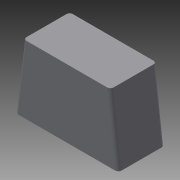
# Autodesk Inventor part: Box MKIV Version 2
Saved by Autodesk Inventor 2013 (Build 170138000, 138)
## iProperties
Created: 2014-12-24
Part Number: Box MKIV Version 2
Material: Generic
Document SubType Name: Modeling
Designer: Zep
Density: 1 g/cm^3
Author: Zep
Autodesk Inventor part; units mm, degrees
ref_plane "YZ Plane" through (0, 0, 0) normal (1, 0, 0) x (0, 1, 0)
ref_plane "XZ Plane" through (0, 0, 0) normal (0, 1, 0) x (-1, 0, 0)
ref_plane "XY Plane" through (0, 0, 0) normal (0, 0, 1) x (1, 0, 0)
sketch "Sketch1" plane through (0, 0, 0) normal (0, 0, 1) x (1, 0, 0)
  line L0 (0, 0) -> (129, 0)
  line L1 (129, 0) -> (129, 85)
  line L2 (129, 85) -> (0, 85)
  line L3 (0, 85) -> (0, 0)
  line L4 (0, 85) -> (10, 85)
  line L5 (10, 85) -> (0, 0)
  line L6 (129, 85) -> (119, 85)
  line L7 (119, 85) -> (129, 0)
  dimension "d0" = 129
  dimension "d1" = 85
  dimension "d2" = 10
  dimension "d3" = 10
  constraints: 16 end point, 2 parallel, 2 point on line, 1 horizontal, 1 perpendicular
  measures "d0" distance of L2.end L1.end
  measures "d1" distance of L1.end L0.end
  measures "d2" distance of L2.end L4.end
  measures "d3" distance of L1.end L6.end
extrude "Extrusion1" add sketch "Sketch1" against normal blind 58 contours L5 L2 L7 L0
fillet "Fillet1" radius 4 4 edges at (5, 42.5, 0) (124, 42.5, 0) (124, 42.5, -58) (5, 42.5, -58)
shell "Shell1" thickness 3 removed faces 1 at (44.3425, 0, -19.3333)
sketch "Sketch3" plane through (0, 0, -58) normal (0, 0, -1) x (-1, 0, 0)
  line L0 (-14.0276, 85) -> (-114.9724, 85) projected
  line L1 (-124.9724, 0) -> (-4.0276, 0) projected
  line L2 (-64.5, 0) -> (-64.5, 85)
  line L3 (-64.5, 85) -> (-64.5, 55)
  circle A0 centre (-64.5, 55) radius 22.5
  line L4 (-64.5, 0) -> (-102.5, 0)
  line L5 (-102.5, 0) -> (-102.5, 20)
  line L6 (-102.5, 20) -> (-64.5, 20)
  line L7 (-64.5, 20) -> (-64.5, 0)
  line L8 (-64.5, 0) -> (-26.5, 0)
  line L9 (-26.5, 0) -> (-26.5, 20)
  line L10 (-26.5, 20) -> (-64.5, 20)
  line L11 (-64.5, 20) -> (-64.5, 0)
  circle A1 centre (-26.5, 20) radius 7.85
  circle A2 centre (-102.5, 20) radius 7.85
  point P0 (0, 0)
  dimension "d18" = 30
  dimension "d19" = 45
  dimension "d20" = 38
  dimension "d21" = 20
  dimension "d22" = 38
  dimension "d23" = 15.7
  dimension "d24" = 15.7
  constraints: 20 end point, 4 parallel, 3 centre point, 3 coincident, 2 horizontal, 2 midpoint, 2 perpendicular, 1 point on line
  measures "d18" distance of L2.end L3.end
  measures "d19" diameter of A0
  measures "d20" distance of L5.end L6.end
  measures "d21" distance of L4.end L5.end
  measures "d22" distance of L10.end L9.end
  measures "d23" diameter of A1
  measures "d24" diameter of A2
extrude "Extrusion3" cut sketch "Sketch3" against normal blind 10 contours A0 L2 | L2 A0 | A2 L6 L5 | L5 L6 A2 | A1 L10 L9 | L9 L10 A1
chamfer "Chamfer1" distance 3 distance2 1 1 edges at (87, 55, -58) measured on face at (52.7612, 4.22, -58)
body "Solid1"
